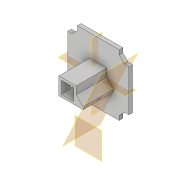
# Autodesk Inventor part: 20_Cube_Insert_Lightsheet_FEPTube_Flowcube_small_v3
Saved by Autodesk Inventor 2022 (Build 260153000, 153)
## iProperties
Created: 2019-07-01
Part Number: 20_Cube_Insert_Lightsheet_FEPTube_Flowcube_small_v3
Material: Generic
Document SubType Name: Modeling
Designer: diederichbenedict
Density: 1 g/cm^3
Appearance: Default
Author: diederichbenedict
Autodesk Inventor part; units mm, degrees
ref_plane "YZ Plane" through (0, 0, 0) normal (1, 0, 0) x (0, 1, 0)
ref_plane "XZ Plane" through (0, 0, 0) normal (0, 1, 0) x (-1, 0, 0)
ref_plane "Work Plane1" through (0, 0, 10) normal (0, 0, 1) x (1, 0, 0)
sketch "Sketch1" plane through (0, 0, 10) normal (0, 0, 1) x (1, 0, 0)
  line L0 (-4.0299, -0.3538) -> (-2.2322, 1.4439) construction
  arc A0 (-1.4439, 2.2322) -> (-2.2322, 1.4439) centre (-0.9299, 0.9299) ccw construction
  line L1 (-1.4439, 2.2322) -> (0.3538, 4.0299) construction
  line L2 (-37.8299, 42.8299) -> (-37.8299, 37.8299) construction
  line L3 (-37.8299, 37.8299) -> (-42.9208, 37.8299) construction
  line L4 (-37.8299, 42.2137) -> (-37.8299, 45.8299) construction
  line L5 (-37.8299, 45.8299) -> (-4.0299, 45.8299) construction
  line L6 (-4.0299, 45.8299) -> (-4.0299, 42.2137) construction
  line L7 (-4.0299, 4.0299) -> (0.3538, 4.0299) projected
  circle A1 centre (-20.9299, 20.9299) radius 17.5 projected
  line L8 (-20.9299, 58.9723) -> (17.1124, 20.9299) construction
  line L9 (17.1124, 20.9299) -> (-20.9299, -17.1124) construction
  line L10 (-20.9299, -17.1124) -> (-58.9723, 20.9299) construction
  line L11 (-58.9723, 20.9299) -> (-20.9299, 58.9723) construction
  line L12 (-20.9299, 58.9723) -> (-20.9299, -17.1124) construction
  line L13 (17.1124, 20.9299) -> (-58.9723, 20.9299) construction
  line L14 (-20.9299, 58.9723) -> (32.8701, 58.9723) construction
  line L15 (-43.4299, 43.4299) -> (1.5701, 43.4299) construction
  line L16 (1.5701, 43.4299) -> (1.5701, -1.5701) construction
  line L17 (1.5701, -1.5701) -> (-43.4299, -1.5701) construction
  line L18 (-43.4299, -1.5701) -> (-43.4299, 43.4299) construction
  line L19 (-43.4299, 43.4299) -> (1.5701, -1.5701) construction
  line L20 (1.5701, 43.4299) -> (-43.4299, -1.5701) construction
  line L21 (-43.4299, 5.3876) -> (-43.4299, 36.4723)
  line L22 (-43.4299, 36.4723) -> (-36.4723, 43.4299)
  line L23 (-36.4723, 43.4299) -> (-5.3876, 43.4299)
  line L24 (-5.3876, 43.4299) -> (1.5701, 36.4723)
  line L25 (1.5701, 36.4723) -> (1.5701, 5.3876)
  line L26 (1.5701, 5.3876) -> (-5.3876, -1.5701)
  line L27 (-5.3876, -1.5701) -> (-36.4723, -1.5701)
  line L28 (-36.4723, -1.5701) -> (-43.4299, 5.3876)
  line L29 (-4.0299, 42.2137) -> (-37.8299, 42.2137) projected
  line L30 (-4.0299, -0.3538) -> (-4.0299, 4.0299) projected
  circle A2 centre (-20.9299, 20.9299) radius 1.5
  line L31 (-10.9299, 10.9299) -> (-30.9299, 10.9299) construction
  line L32 (-30.9299, 10.9299) -> (-30.9299, 30.9299) construction
  line L33 (-30.9299, 30.9299) -> (-10.9299, 30.9299) construction
  line L34 (-10.9299, 30.9299) -> (-10.9299, 10.9299) construction
  line L35 (-10.9299, 10.9299) -> (-30.9299, 30.9299) construction
  line L36 (-30.9299, 10.9299) -> (-10.9299, 30.9299) construction
  circle A3 centre (-30.9299, 30.9299) radius 1.4
  circle A4 centre (-30.9299, 10.9299) radius 1.4
  circle A5 centre (-10.9299, 10.9299) radius 1.4
  line L37 (-45.8299, 37.8299) -> (-42.0723, 37.8299) construction
  line L38 (-42.1723, 37.7299) -> (-45.8299, 37.7299)
  line L39 (-45.8299, 37.7299) -> (-45.8299, 4.1299)
  line L40 (-45.8299, 4.1299) -> (-42.1723, 4.1299)
  line L41 (-42.1723, 4.1299) -> (-42.1723, 37.7299)
  line L42 (-45.8299, 4.0299) -> (-42.0723, 4.0299) construction
  line L43 (-45.8299, 37.8299) -> (-42.0723, 37.8299) projected
  line L44 (-37.7299, 45.8299) -> (-4.1299, 45.8299)
  line L45 (-4.1299, 45.8299) -> (-4.1299, 42.1723)
  line L46 (-4.1299, 42.1723) -> (-37.7299, 42.1723)
  line L47 (-37.7299, 42.1723) -> (-37.7299, 45.8299)
  line L48 (0.4701, 37.8299) -> (0.4701, 4.0299) construction
  line L49 (0.4701, 4.0299) -> (3.9701, 4.0299) construction
  line L50 (3.9701, 37.8299) -> (3.9701, 4.0299) construction
  line L51 (0.4701, 37.8299) -> (3.9701, 37.8299) construction
  line L52 (-45.8299, -3.9701) -> (-4.0299, -3.9701) construction
  line L53 (0.3124, 37.7299) -> (3.9701, 37.7299)
  line L54 (3.9701, 37.7299) -> (3.9701, 4.1299)
  line L55 (3.9701, 4.1299) -> (0.3124, 4.1299)
  line L56 (0.3124, 4.1299) -> (0.3124, 37.7299)
  line L57 (-4.1713, -0.3538) -> (-37.7299, -0.3538)
  line L58 (-37.7299, -0.3538) -> (-37.7299, -3.9701)
  line L59 (-37.7299, -3.9701) -> (-4.1713, -3.9701)
  line L60 (-4.1713, -3.9701) -> (-4.1713, -0.3538)
  point P0 (-37.8299, 4.0299)
  dimension "d18" = 53.8
  dimension "d19" = 45
  dimension "d20" = 53.8
  dimension "d21" = 45
  dimension "d22" = 45
  dimension "d30" = 20
  dimension "d31" = 20
  dimension "d32" = 2.8
  dimension "d33" = 2.8
  dimension "d34" = 2.8
  dimension "d35" = 3
  dimension "d36" = 0.1
  dimension "d37" = 0.1
  dimension "d38" = 0.1
  dimension "d39" = 0.1
  constraints: 86 end point, 21 point on line, 14 parallel, 8 perpendicular, 7 horizontal, 7 midpoint, 4 centre point, 4 coincident, 1 equal length
  measures "d18" distance of L8.start L8.end
  measures "d19" angle of L8 L14
  measures "d20" distance of L8.end L9.end
  measures "d21" distance of L16.end L17.end
  measures "d22" distance of L15.end L16.end
  measures "d30" distance of L32.end L33.end
  measures "d31" distance of L31.end L32.end
  measures "d32" diameter of A3
  measures "d33" diameter of A4
  measures "d34" diameter of A5
  measures "d35" diameter of A2
  measures "d36" distance between parallel lines of L38 L43
  measures "d37" distance between parallel lines of L40 L42
  measures "d38" distance between parallel lines of L45 L6
  measures "d39" distance between parallel lines of L4 L47
extrude "Extrusion1" add sketch "Sketch1" along normal blind 3 contours L30 L26 L57 L28 L41 L22 L46 L24 L56 L7 | L7 L26 L30 | L56 L24 L25 L26 | L26 L25 L24 L53 L54 L55 | L60 L59 L58 L57 L28 L27 L26 | L26 L27 L28 L57 | L46 L22 L29 L24 | L24 L29 L45 | L40 L39 L38 L22 L21 L28 | L28 L21 L22 L41 | L29 L22 L23 L24 | L24 L23 L22 L29 L47 L44 L45 | L47 L29 L22 | A1 | A2 | A3 | A4 | A5
sketch "Skizze4" plane through (0, 0, 13) normal (0, 0, 1) x (1, 0, 0)
  line L0 (-37.7299, 42.1723) -> (-42.1723, 37.7299) projected
  line L1 (-42.1723, 37.7299) -> (-45.8299, 37.7299) projected
  line L2 (-45.8299, 37.7299) -> (-45.8299, 4.1299) construction
  line L3 (-45.8299, 4.1299) -> (-42.1723, 4.1299) projected
  line L4 (-42.1723, 4.1299) -> (-37.6885, -0.3538) projected
  line L5 (-37.6885, -0.3538) -> (-37.7299, -0.3538) projected
  line L6 (-37.7299, -0.3538) -> (-37.7299, -3.9701) projected
  line L7 (-37.7299, -3.9701) -> (-4.1713, -3.9701) construction
  line L8 (-4.1713, -3.9701) -> (-4.1713, -0.3538) projected
  line L9 (-4.1713, -0.3538) -> (0.3124, 4.1299) projected
  line L10 (0.3124, 4.1299) -> (3.9701, 4.1299) projected
  line L11 (3.9701, 4.1299) -> (3.9701, 37.7299) construction
  line L12 (3.9701, 37.7299) -> (0.3124, 37.7299) projected
  line L13 (0.3124, 37.7299) -> (-4.1299, 42.1723) projected
  line L14 (-4.1299, 42.1723) -> (-4.1299, 45.8299) projected
  line L15 (-4.1299, 45.8299) -> (-37.7299, 45.8299) construction
  line L16 (-37.7299, 45.8299) -> (-37.7299, 42.1723) projected
  line L17 (-37.9299, 46.0299) -> (-3.9299, 46.0299) construction
  line L18 (-3.9299, 46.0299) -> (-3.9299, 42.2551)
  line L19 (-3.9299, 42.2551) -> (0.3953, 37.9299)
  line L20 (0.3953, 37.9299) -> (4.1701, 37.9299)
  line L21 (4.1701, 37.9299) -> (4.1701, 3.9299) construction
  line L22 (4.1701, 3.9299) -> (0.3953, 3.9299)
  line L23 (0.3953, 3.9299) -> (-3.9713, -0.4367)
  line L24 (-3.9713, -0.4367) -> (-3.9713, -4.1701)
  line L25 (-3.9713, -4.1701) -> (-37.9299, -4.1701) construction
  line L26 (-37.9299, -4.1701) -> (-37.9299, -0.3953)
  line L27 (-37.9299, -0.3953) -> (-42.2551, 3.9299)
  line L28 (-42.2551, 3.9299) -> (-46.0299, 3.9299)
  line L29 (-46.0299, 3.9299) -> (-46.0299, 37.9299) construction
  line L30 (-46.0299, 37.9299) -> (-42.2551, 37.9299)
  line L31 (-42.2551, 37.9299) -> (-37.9299, 42.2551)
  line L32 (-37.9299, 42.2551) -> (-37.9299, 46.0299)
  line L33 (-45.8299, 37.7299) -> (-45.8299, 37.9299)
  line L34 (-4.1299, 45.8299) -> (-37.7299, 45.8299) projected
  line L35 (-37.7299, 45.8299) -> (-37.9299, 45.8299)
  line L36 (-4.1299, 45.8299) -> (-3.9299, 45.8299)
  line L37 (3.9701, 37.7299) -> (3.9701, 37.9299)
  line L38 (3.9701, 4.1299) -> (3.9701, 37.7299) projected
  line L39 (3.9701, 4.1299) -> (3.9701, 3.9299)
  line L40 (-4.1713, -3.9701) -> (-3.9713, -3.9701)
  line L41 (-37.7299, -3.9701) -> (-37.9299, -3.9701)
  line L42 (-45.8299, 4.1299) -> (-45.8299, 3.9299)
  point P0 (0, 0)
  dimension "d40" = 0.2
  constraints: 48 end point, 12 point on line, 4 perpendicular, 15 other
  measures "d40" distance between parallel lines of L15 L17
extrude "IM_offset" add sketch "Skizze4" against normal up to surface (3 mm away)
ref_plane "Arbeitsebene5" through (-20.9299, 3.9299, 10) normal (1, 0, 0) x (0, 0, -1)
ref_plane "Arbeitsebene6" through (-37.9299, 20.9299, 10) normal (0, 1, 0) x (1, 0, 0)
sketch "Skizze25" plane through (0, 0, 13) normal (0, 0, 1) x (1, 0, 0)
  line L0 (3.9701, 3.9299) -> (3.9701, 37.9299) projected
  line L1 (3.9701, 37.9299) -> (0.3953, 37.9299) projected
  line L2 (0.3953, 37.9299) -> (-3.9299, 42.2551) projected
  line L3 (-3.9299, 42.2551) -> (-3.9299, 45.8299) projected
  line L4 (-3.9299, 45.8299) -> (-37.9299, 45.8299) projected
  line L5 (-37.9299, 45.8299) -> (-37.9299, 42.2551) projected
  line L6 (-37.9299, 42.2551) -> (-42.2551, 37.9299) projected
  line L7 (-42.2551, 37.9299) -> (-45.8299, 37.9299) projected
  line L8 (-45.8299, 37.9299) -> (-45.8299, 3.9299) projected
  line L9 (-42.2551, 3.9299) -> (-45.8299, 3.9299) projected
  line L10 (-37.9299, -0.3953) -> (-42.2551, 3.9299) projected
  line L11 (-37.9299, -3.9701) -> (-37.9299, -0.3953) projected
  line L12 (-3.9713, -3.9701) -> (-37.9299, -3.9701) projected
  line L13 (-3.9713, -3.9701) -> (-3.9713, -0.4367) projected
  line L14 (-3.9713, -0.4367) -> (0.3953, 3.9299) projected
  line L15 (0.3953, 3.9299) -> (3.9701, 3.9299) projected
  line L16 (-11.384, 9.2627) -> (-32.5972, 30.4759)
  line L17 (-15.9506, 25.9092) -> (-25.9506, 25.9092)
  line L18 (-25.9506, 25.9092) -> (-25.9506, 15.9092)
  line L19 (-25.9506, 15.9092) -> (-15.9506, 15.9092)
  line L20 (-15.9506, 15.9092) -> (-15.9506, 25.9092)
  line L21 (-15.9506, 25.9092) -> (-25.9506, 15.9092) construction
  line L22 (-25.9506, 25.9092) -> (-15.9506, 15.9092) construction
  line L23 (-13.9506, 27.9092) -> (-27.9506, 27.9092)
  line L24 (-27.9506, 27.9092) -> (-27.9506, 13.9092)
  line L25 (-27.9506, 13.9092) -> (-13.9506, 13.9092)
  line L26 (-13.9506, 13.9092) -> (-13.9506, 27.9092)
  line L27 (-15.9506, 20.9092) -> (-13.9506, 20.9092)
  line L28 (-20.9506, 25.9092) -> (-20.9506, 27.9092)
  line L29 (-18.0305, 15.9092) -> (-15.9506, 18.072)
  line L30 (-25.9506, 23.8293) -> (-23.7879, 25.9092)
  line L31 (-27.9506, 27.9092) -> (-25.9506, 27.9092)
  line L32 (-13.9506, 13.9092) -> (-8.2901, 13.9092)
  line L33 (-8.2901, 13.9092) -> (-8.2901, 15.9092)
  line L34 (-8.2901, 15.9092) -> (-13.9506, 15.9092)
  line L35 (-13.9506, 15.9092) -> (-13.9506, 13.9092)
  line L36 (-8.2901, 15.9092) -> (-13.9506, 21.5697)
  point P0 (0, 0)
  point P1 (-20.9506, 20.9092)
  point P2 (-13.9506, 15.9092)
  dimension "d150" = 10
  dimension "d151" = 10
  dimension "d152" = 2
  dimension "d154" = 7
  constraints: 43 end point, 7 point on line, 6 midpoint, 6 parallel, 4 horizontal, 4 perpendicular, 6 other
  measures "d150" distance of L19.end L18.end
  measures "d151" distance of L18.end L17.end
  measures "d152" distance between parallel lines of L20 L26
  measures "d154" distance between parallel lines of L25 L27
extrude "Extrusion21" add sketch "Skizze25" along normal blind 25 contours L19 L20 L27 L26 L25 L16 | L16 L25 L24 L18 L19 | L16 L24 L23 L28 L17 L18 | L26 L34 L33 L32 | L20 L17 L28 L23 L26 L27 | L26 L36 L34
ref_plane "Arbeitsebene10" through (0, 0, 42) normal (0, 0, 1) x (1, 0, 0)
ref_plane "Arbeitsebene9" through (-28.9506, 12.9092, 13) normal (-1, 0, 0) x (0, 0, 1)
sketch "Skizze28" plane through (-28.9506, 12.9092, 13) normal (-1, 0, 0) x (0, 0, 1)
  line L0 (0, 3) -> (0, 13) projected
  line L1 (0, 3) -> (25, 3) projected
  line L2 (25, 13) -> (25, 3) projected
  line L3 (0, 13) -> (25, 13) projected
  line L4 (17.5, 3) -> (7.5, 3)
  line L5 (7.5, 3) -> (7.5, 6)
  line L6 (7.5, 6) -> (17.5, 6)
  line L7 (17.5, 6) -> (17.5, 3)
  line L8 (17.5, 3) -> (7.5, 6) construction
  line L9 (7.5, 3) -> (17.5, 6) construction
  point P0 (-13, -12.9092)
  point P1 (12.5, 4.5)
  point P2 (17.5, 3)
  point P3 (17.5, 13)
  point P4 (7.5, 13)
  dimension "d187" = 10
  dimension "d188" = 3
  constraints: 12 end point, 2 midpoint, 2 parallel, 1 horizontal, 1 perpendicular, 1 point on line
  measures "d187" distance of L5.end L6.end
  measures "d188" distance of L4.end L5.end
extrude "Extrusion24" cut sketch "Skizze28" against normal blind 3 contours L5 L6 L7 L1
sketch "Skizze34" plane through (-27.9506, 13.9092, 13) normal (0, -1, 0) x (1, 0, 0)
  line L0 (19.6605, 0) -> (0, 0) projected
  line L1 (19.6605, 0) -> (19.6605, 25) projected
  line L2 (0, 25) -> (19.6605, 25) projected
  line L3 (0, 0) -> (0, 25) projected
  circle A0 centre (8.0421, 12.5) radius 5.5
  point P0 (27.9506, -13)
  dimension "d192" = 11
  constraints: 1 centre point
  measures "d192" diameter of A0
extrude "Extrusion30" cut sketch "Skizze34" against normal blind 3 contours A0
sketch "Skizze35" plane through (-27.9506, 13.9092, 13) normal (0, -1, 0) x (1, 0, 0)
  circle A0 centre (8.0421, 12.5) radius 5.5 projected
  circle A1 centre (8.0421, 12.5) radius 6.5
  point P0 (27.9506, -13)
  dimension "d195" = 13
  constraints: 1 centre point, 1 coincident
  measures "d195" diameter of A1
extrude "Extrusion31" cut sketch "Skizze35" against normal blind 1 contours A0 | A1
sketch "Skizze36" plane through (-27.9506, 13.9092, 13) normal (-1, 0, 0) x (0, 0, 1)
  circle A0 centre (12.5608, 1.7467) radius 6.5
  point P0 (-13, -13.9092)
  dimension "d202" = 13
  constraints: 1 centre point
  measures "d202" diameter of A0
extrude "Extrusion32" cut sketch "Skizze36" against normal blind 1
ref_plane "Arbeitsebene12" through (-8.2901, 13.9092, 13) normal (0.9063, -0.4226, 0) x (0, 0, 1)
sketch "Skizze37" plane through (-8.2901, 13.9092, 13) normal (0.9063, -0.4226, 0) x (0, 0, 1)
  circle A0 centre (12.5, -0.6497) radius 1
  ellipse E0 centre (12.5, 4.9101) end of major axis (6, 4.9101) minor radius 2.747 projected
  point P0 (-13, 9.1025)
  dimension "d204" = 2
  constraints: 1 centre point, 1 other
  measures "d204" diameter of A0
extrude "Extrusion33" cut sketch "Skizze37" against normal through all contours A0
body "Solid1"
